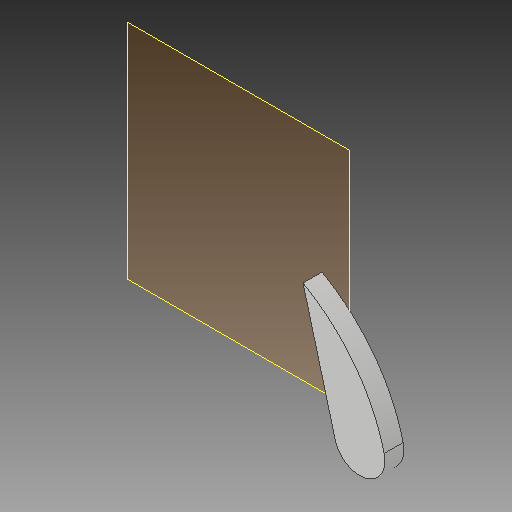
# Autodesk Inventor part: Part12
Saved by Autodesk Inventor 2017 (Build 210142000, 142)
## iProperties
Created: 2017-01-16
Part Number: Part12
Material: Generic
Document SubType Name: Modeling
Designer: mmarkle
Density: 1 g/cm^3
Appearance: Default
Author: mmarkle
Autodesk Inventor part; units mm, degrees
ref_plane "YZ Plane" through (0, 0, 0) normal (1, 0, 0) x (0, 1, 0)
ref_plane "XZ Plane" through (0, 0, 0) normal (0, 1, 0) x (-1, 0, 0)
ref_plane "XY Plane" through (0, 0, 0) normal (0, 0, 1) x (1, 0, 0)
ref_plane "Work Plane1" through (0, 0, 0) normal (0, 0, 1) x (1, 0, 0)
sketch "Sketch1" plane through (0, 0, 0) normal (0, 0, 1) x (1, 0, 0)
  arc A0 (29.0656, -32.0182) -> (41.3613, -28.8418) centre (35.1974, -30.368) ccw
  line L0 (20.9812, -1.9785) -> (29.0656, -32.0182)
  arc A1 (41.3613, -28.8418) -> (20.9812, -1.9785) centre (-0.0479, -39.0948) ccw
  point P0 (0, 0)
  dimension "d0" = 31.75
  dimension "d1" = 12.7
  constraints: 4 point on circle, 2 centre point, 2 end point, 2 tangent
  measures "d0" distance of L0.start A0.centre
  measures "d1" diameter of A0
extrude "Extrusion1" add sketch "Sketch1" along normal blind 4.7625
body "Solid1"
